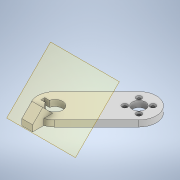
# Autodesk Inventor part: Pièce_moteur_maintient_test_8
Saved by Autodesk Inventor 2020.1 (Build 241239000, 239)
## iProperties
Created: 2019-07-26
Part Number: Pièce_moteur_maintient_test_8
Material: Générique
Document SubType Name: Modeling
Designer: marlo
Density: 1 g/cm^3
Appearance: Par défaut
Author: marlo
Autodesk Inventor part; units mm, degrees
ref_plane "YZ Plane" through (0, 0, 0) normal (1, 0, 0) x (0, 1, 0)
ref_plane "XZ Plane" through (0, 0, 0) normal (0, 1, 0) x (-1, 0, 0)
ref_plane "XY Plane" through (0, 0, 0) normal (0, 0, 1) x (1, 0, 0)
sketch "Esquisse3" plane through (0, 0, 0) normal (0, 1, 0) x (-1, 0, 0)
  line L0 (-4.7436, 8.0343) -> (8.2564, 8.0343) construction
  line L1 (8.2564, 8.0343) -> (8.2564, -4.9657) construction
  line L2 (8.2564, -4.9657) -> (-4.7436, -4.9657) construction
  line L3 (-4.7436, -4.9657) -> (-4.7436, 8.0343) construction
  line L4 (-4.7436, 8.0343) -> (8.2564, -4.9657) construction
  line L5 (8.2564, 8.0343) -> (-4.7436, -4.9657) construction
  line L6 (-9.9657, 13.2564) -> (13.2564, 13.2564) construction
  line L7 (13.2564, 13.2564) -> (13.2564, -9.9657) construction
  line L8 (13.2564, -9.9657) -> (-9.9657, -9.9657) construction
  line L9 (-9.9657, -9.9657) -> (-9.9657, 13.2564) construction
  line L10 (-9.9657, 13.2564) -> (13.2564, -9.9657) construction
  line L11 (13.2564, 13.2564) -> (-9.9657, -9.9657) construction
  line L12 (-4.7436, 8.0343) -> (-9.9657, 8.0343) construction
  line L13 (-9.9657, 8.0343) -> (-9.9657, 13.2564) construction
  line L14 (-9.9657, 13.2564) -> (-4.7436, 13.2564) construction
  line L15 (-4.7436, 13.2564) -> (-4.7436, 8.0343) construction
  line L16 (-4.7436, -4.9657) -> (-9.9657, -4.9657) construction
  line L17 (-9.9657, -4.9657) -> (-9.9657, -9.9657) construction
  line L18 (-9.9657, -9.9657) -> (-4.7436, -9.9657) construction
  line L19 (-4.7436, -9.9657) -> (-4.7436, -4.9657) construction
  line L20 (8.2564, -4.9657) -> (13.2564, -4.9657) construction
  line L21 (13.2564, -4.9657) -> (13.2564, -9.9657) construction
  line L22 (13.2564, -9.9657) -> (8.2564, -9.9657) construction
  line L23 (8.2564, -9.9657) -> (8.2564, -4.9657) construction
  line L24 (13.2564, 13.2564) -> (8.2564, 13.2564) construction
  line L25 (8.2564, 13.2564) -> (8.2564, 8.0343) construction
  line L26 (8.2564, 8.0343) -> (13.2564, 8.0343) construction
  line L27 (13.2564, 8.0343) -> (13.2564, 13.2564) construction
  circle A0 centre (10.8675, 10.6453) radius 2.6111
  circle A1 centre (10.7564, -7.4657) radius 2.5
  circle A2 centre (-7.3547, -7.5768) radius 2.6111
  circle A3 centre (-7.3547, 10.6453) radius 2.6111
  circle A4 centre (1.7564, 1.5343) radius 22.5
  circle A5 centre (1.7564, 1.5343) radius 8.5
  circle A6 centre (56.2036, 55.9815) radius 22.5
  circle A7 centre (56.2036, 55.9815) radius 10
  line L28 (58.2036, 65.7795) -> (54.2036, 65.7795)
  line L29 (54.2036, 65.7795) -> (54.2036, 86.7795)
  line L30 (54.2036, 86.7795) -> (58.2036, 86.7795)
  line L31 (58.2036, 86.7795) -> (58.2036, 65.7795)
  line L32 (49.2036, 91.7795) -> (49.2036, 60.7795)
  line L33 (49.2036, 60.7795) -> (63.2036, 60.7795)
  line L34 (63.2036, 60.7795) -> (63.2036, 91.7795)
  line L35 (63.2036, 91.7795) -> (49.2036, 91.7795)
  line L36 (71.8861, 53.4815) -> (65.8861, 53.4815)
  line L37 (65.8861, 53.4815) -> (65.8861, 58.4815)
  line L38 (65.8861, 58.4815) -> (71.8861, 58.4815)
  line L39 (71.8861, 58.4815) -> (71.8861, 53.4815)
  line L40 (17.6663, -14.3756) -> (-14.1535, 17.4442) construction
  line L41 (17.6663, -14.3756) -> (72.1135, 40.0716)
  line L42 (-14.1535, 17.4442) -> (40.2937, 71.8914)
  line L43 (-14.1535, -14.3756) -> (72.1135, 71.8914) construction
  point P0 (1.7564, 1.5343)
  point P1 (10.5343, 10.5343)
  point P2 (78.7036, 55.9815)
  point P3 (17.4356, 66.5)
  point P4 (63.2036, 77.3649)
  point P5 (49.2036, 77.3649)
  point P6 (58.2036, 78.3924)
  point P7 (54.2036, 78.3924)
  point P8 (49.2036, 63.1229)
  point P9 (63.2036, 63.1229)
  dimension "d1" = 13
  dimension "d2" = 13
  dimension "d3" = 5
  dimension "d4" = 45
  dimension "d31" = 45
  dimension "d32" = 20
  dimension "d33" = 4
  dimension "d34" = 21
  dimension "d36" = 5
  dimension "d37" = 5
  dimension "d51" = 6
  dimension "d56" = 122
  dimension "d62" = 17
  constraints: 88 end point, 20 parallel, 12 tangent, 11 point on circle, 9 perpendicular, 8 centre point, 8 horizontal, 6 coincident, 4 collinear, 2 midpoint, 2 point on line, 3 other
  measures "d1" distance of L0.end L1.end
  measures "d2" distance of L0.start L0.end
  measures "d3" distance between parallel lines of L2 L8
  measures "d4" diameter of A4
  measures "d31" diameter of A6
  measures "d32" diameter of A7
  measures "d33" distance of L29.end L30.end
  measures "d34" distance of L30.end L28.start
  measures "d36" distance between parallel lines of L29 L32
  measures "d37" distance of L38.end L36.start
  measures "d51" distance of L36.start L36.end
  measures "d56" distance of L43.start L43.end
  measures "d62" diameter of A5
extrude "Extrusion1" add sketch "Esquisse3" along normal blind 8 contours A4 | A4 L42 A6 L41 | A6 L32 A7 L36 L39 L38 L34 | L32 L35 L34 A6 L31 L30 L29 | A6 L29 A7 L32 | L34 A7 L31 A6
chamfer "Chanfrein5" distance 1 distance2 2 1 edges at (9.9657, 8, -7.5768) measured on face at (10.4657, 8, -7.5768)
chamfer "Chanfrein6" distance 1 distance2 2 1 edges at (-8.2564, 8, -7.4657) measured on face at (-7.7564, 8, -7.4657)
chamfer "Chanfrein7" distance 1 distance2 2 1 edges at (-8.2564, 8, 10.6453) measured on face at (-7.7564, 8, 10.6453)
chamfer "Chanfrein8" distance 1 distance2 2 1 edges at (9.9657, 8, 10.6453) measured on face at (10.4657, 8, 10.6453)
ref_plane "Plan de construction1" through (-63.2036, 8, 91.7795) normal (0, 0.7071068, 0.7071068) x (1, 0, 0)
sketch "Esquisse8" plane through (-63.2036, 8, 91.7795) normal (0, 0.7071068, 0.7071068) x (1, 0, 0)
  line L0 (0, 4.5358) -> (0, -5.6569) projected
  line L1 (0, 0) -> (14, 0)
  line L2 (14, 0) -> (14, 18.3465)
  line L3 (14, 18.3465) -> (0, 18.3465)
  line L4 (0, 18.3465) -> (0, 0)
  line L5 (9, 3.5355) -> (5, 3.5355) projected
  line L6 (9, 3.5355) -> (5, 3.5355)
  line L7 (5, 3.5355) -> (5, 18.3465)
  line L8 (5, 18.3465) -> (9, 18.3465)
  line L9 (9, 18.3465) -> (9, 3.5355)
  line L10 (14, 0) -> (14, 10.1926) projected
  line L11 (5, 3.5355) -> (5, 18.3848) projected
  point P0 (63.2036, 59.241)
  point P1 (9, 18.3465)
  point P2 (5, 3.5355)
  constraints: 16 end point, 4 parallel, 2 collinear, 2 horizontal, 2 perpendicular, 2 point on line
extrude "Extrusion3" add sketch "Esquisse8" against normal up to surface contours L4 L3 L7 L5 L9 L2 L1 L0 surface through (-1.7564, 8, 1.5343) normal (0, 1, 0)
sketch "Esquisse9" plane through (-54.2036, 10.5, 89.2795) normal (0, 0.7071068, -0.7071068) x (-1, 0, 0)
  line L0 (0, -3.5355) -> (4, -3.5355) projected
  line L1 (0, -3.5355) -> (4, -3.5355)
  line L2 (4, -3.5355) -> (4, 0)
  line L3 (4, 0) -> (0, 0)
  line L4 (0, 0) -> (0, -3.5355)
  line L5 (4, 0) -> (4, -18.3465) projected
  point P0 (-54.2036, -70.5547)
  constraints: 8 end point, 2 parallel, 1 collinear, 1 horizontal, 1 perpendicular
extrude "Extrusion4" add sketch "Esquisse9" along normal up to surface (14.811 mm away)
